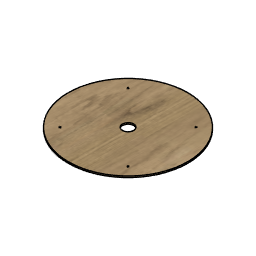
Top Plane (Autodesk Fusion 360 design; units mm, degrees)
Autodesk Fusion 360 part; units mm, degrees
sketch "Sketch1" plane through (0, 0, 0) normal (0, 0, 1) x (1, 0, 0)
  circle A0 centre (-75, 75) radius 1.75
  circle A1 centre (-75, -75) radius 1.75
  circle A2 centre (75, -75) radius 1.75
  circle A3 centre (75, 75) radius 1.75
  circle A4 centre (0, 0) radius 132
  circle A5 centre (0, 0) radius 12.5
  dimension "d1" = 264
  dimension "d4" = 3.5
  dimension "d6" = 360
  dimension "d46" = 75
  dimension "d47" = 75
  dimension "d48" = 25
  constraint coincident A4.centre A5.centre
  constraint concentric A4 A5
  measures "d1" diameter of A4
  measures "d4" diameter of A0
  measures "d46" horizontal distance of A4.centre A0.centre
  measures "d47" vertical distance of A4.centre A0.centre
  measures "d48" diameter of A5
extrude "Extrude1" add sketch "Sketch1" along normal blind 3
